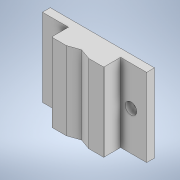
# Autodesk Inventor part: Soporte Superior Tubos
Saved by Autodesk Inventor 2021 (Build 250183000, 183)
## iProperties
Created: 2021-05-02
Part Number: Soporte Superior Tubos
Material: Generic
Document SubType Name: Modeling
Designer: maaro
Density: 1 g/cm^3
Appearance: Default
Author: maaro
Autodesk Inventor part; units mm, degrees
ref_plane "YZ Plane" through (0, 0, 0) normal (1, 0, 0) x (0, 1, 0)
ref_plane "XZ Plane" through (0, 0, 0) normal (0, 1, 0) x (-1, 0, 0)
ref_plane "XY Plane" through (0, 0, 0) normal (0, 0, 1) x (1, 0, 0)
sketch "Sketch2" plane through (0, 0, 0) normal (0, 0, 1) x (1, 0, 0)
  line L0 (0, 0) -> (200, 0)
  line L1 (200, 0) -> (200, 150)
  line L2 (200, 150) -> (0, 150)
  line L3 (0, 150) -> (0, 0)
  dimension "d4" = 150
  dimension "d5" = 200
  constraints: 8 end point, 2 parallel, 1 horizontal, 1 perpendicular
  measures "d4" distance of L2.end L0.start
  measures "d5" distance of L1.end L2.end
extrude "Extrusion2" add sketch "Sketch2" against normal blind 15
sketch "Sketch3" plane through (0, 0, 0) normal (0, 0, 1) x (1, 0, 0)
  line L0 (200, 150) -> (0, 150) projected
  line L1 (0, 150) -> (0, 0) projected
  point P0 (30, 75)
  point P1 (170, 75)
  dimension "d11" = 75
  dimension "d12" = 75
  dimension "d13" = 140
  dimension "d14" = 30
  measures "d11" distance from line of point (30, 75) L0
  measures "d12" distance from line of point (170, 75) L0
  measures "d13" distance of point (170, 75) point (30, 75)
  measures "d14" distance from line of point (30, 75) L1
hole "Hole1" at (30, 75, 0) at (170, 75, 0) direction (0, 0, -1) diameter 22.05 end through all
sketch "Sketch6" plane through (0, 150, 0) normal (0, 1, 0) x (1, 0, 0)
  line L0 (0, 0) -> (200, 0) projected
  line L1 (50, 0) -> (150, 0)
  line L2 (150, 0) -> (150, -32.5)
  line L3 (50, -32.5) -> (50, 0)
  line L4 (0, 0) -> (0, 15) projected
  line L5 (150, -32.5) -> (121.618, -32.5)
  line L6 (121.618, -32.5) -> (100, -25)
  line L7 (100, -25) -> (78.382, -32.5)
  line L8 (78.382, -32.5) -> (50, -32.5)
  dimension "d36" = 50
  dimension "d37" = 100
  dimension "d42" = 32.5
  dimension "d45" = 28.382
  dimension "d46" = 25
  constraints: 14 end point, 3 equal length, 3 point on line, 1 collinear, 1 horizontal, 1 vertical
  measures "d36" distance between parallel lines of L3 L4
  measures "d37" distance between parallel lines of L2 L3
  measures "d42" distance of L1.end L2.end
  measures "d45" distance of L2.end L5.end
  measures "d46" distance from line of L0 L6.end
extrude "Extrusion3" add sketch "Sketch6" against normal blind 150
chamfer "Chamfer1" distance 1 angle 45 2 edges at (150, 75, 32.5) (50, 75, 32.5)
sketch "Sketch7" plane through (0, 0, -15) normal (0, 0, -1) x (-1, 0, 0)
  line L0 (-100, 150) -> (-100, 0) projected
  line L1 (-200, 0) -> (0, 0) projected
  line L2 (0, 0) -> (0, 150) projected
  point P0 (-100, 75)
  dimension "d54" = 75
  dimension "d55" = 100
  constraints: 1 midpoint
  measures "d54" distance from line of L1 point (-100, 75)
  measures "d55" distance from line of L2 point (-100, 75)
hole "Hole3" at (100, 75, -15) direction (0, 0, 1) diameter 8.647 depth 25 tip angle 137 thread size "M10x1.25" class "6H" standard "ISO Metric profile"
equation "\"d12\" = d11"
body "Solid2"
